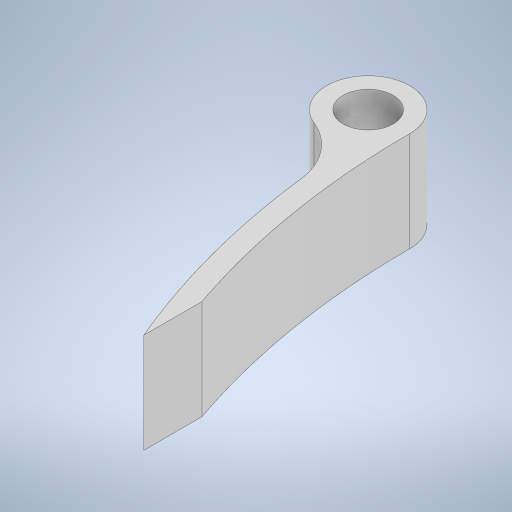
# Autodesk Inventor part: clamp
Saved by Autodesk Inventor 2023 (Build 270158000, 158)
## iProperties
Created: 2024-06-24
Part Number: clamp
Material: Generic
Document SubType Name: Modeling
Designer: Swoby
Density: 1 g/cm^3
Appearance: Default
Author: Swoby
Autodesk Inventor part; units mm, degrees
ref_plane "YZ Plane" through (0, 0, 0) normal (1, 0, 0) x (0, 1, 0)
ref_plane "XZ Plane" through (0, 0, 0) normal (0, 1, 0) x (-1, 0, 0)
ref_plane "XY Plane" through (0, 0, 0) normal (0, 0, 1) x (1, 0, 0)
sketch "Sketch1" plane through (0, 0, 0) normal (0, 1, 0) x (-1, 0, 0)
  circle A0 centre (0, 0) radius 3
  circle A1 centre (0, 0) radius 5
  line L0 (-10.0001, 41) -> (-10, 19) construction
  arc A2 (-5, 0) -> (-10.0001, 30) centre (-97.4989, 0) ccw
  line L1 (0, 0) -> (-5, 0) construction
  line L2 (-10.0001, 30) -> (-10.0001, 37)
  arc A3 (-2.5927, 4.225) -> (-3.1699, 11.2732) centre (-97.4989, 0) ccw construction
  arc A4 (-3.1699, 11.2732) -> (1.8911, 4.6286) centre (5.0052, 12.2502) ccw
  arc A5 (-3.1699, 11.2732) -> (-10.0001, 37) centre (-97.4989, 0) ccw
  dimension "d0" = 6
  dimension "d1" = 2
  dimension "d2" = 10
  dimension "d3" = 30
  dimension "d4" = 5.0001
  dimension "d5" = 7
  constraints: 10 point on circle, 6 centre point, 6 end point, 3 tangent, 1 coincident, 1 horizontal, 1 midpoint, 1 point on line
  measures "d0" diameter of A0
  measures "d1" radial gap between concentric circles of A0 A1
  measures "d2" distance from line of L0 point (0, 0)
  measures "d3" vertical distance of point (0, 0) L2.start
  measures "d4" horizontal distance of L1.end L2.start
  measures "d5" distance of L2.end L2.start
extrude "Extrusion1" add sketch "Sketch1" along normal blind 12
body "Solid1"
